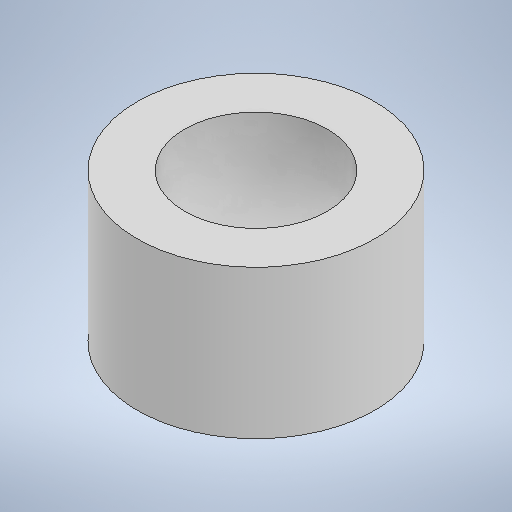
# Autodesk Inventor part: Test1
Saved by Autodesk Inventor 2026.2 (Build 302298010, 298A)
## iProperties
Created: 2026-05-09
Part Number: Test1
Material: Generic
Document SubType Name: Modeling
Designer: piete
Density: 1 g/cm^3
Appearance: Default
Author: piete
Autodesk Inventor part; units mm, degrees
ref_plane "YZ Plane" through (0, 0, 0) normal (1, 0, 0) x (0, 1, 0)
ref_plane "XZ Plane" through (0, 0, 0) normal (0, 1, 0) x (-1, 0, 0)
ref_plane "XY Plane" through (0, 0, 0) normal (0, 0, 1) x (1, 0, 0)
sketch "Sketch1" plane through (0, 0, 0) normal (0, 1, 0) x (-1, 0, 0)
  circle A0 centre (0, 0) radius 20
  dimension "d0" = 40
  constraints: 1 centre point, 1 coincident
  measures "d0" diameter of A0
extrude "Extrusion1" add sketch "Sketch1" along normal blind 25
sketch "Sketch2" plane through (0, 0, 0) normal (1, 0, 0) x (0, 1, 0)
  line L0 (25, -20) -> (25, 20) projected
  line L1 (25, 0) -> (25, -12)
  line L2 (25, -12) -> (25, 12)
  circle A0 centre (25, 12) radius 12.5
  circle A1 centre (25, -12) radius 12.5
  circle A2 centre (21.5, 0) radius 12.5
  line L3 (39.3814, 0) -> (3.1668, 0)
  line L4 (-7.8763, 0) -> (47.2577, 0) projected
  point P0 (0, 0)
  point P1 (34, 0)
  point P2 (9, 0)
  dimension "d5" = 25
  dimension "d6" = 25
  dimension "d3" = 12
  dimension "d4" = 24
  dimension "d7" = 25
  dimension "d8" = 36.2146
  dimension "d9" = 3.1668
  dimension "d10" = 12
  constraints: 6 end point, 2 coincident, 2 point on line, 1 centre point, 1 horizontal, 1 midpoint, 6 other
  measures "d3" distance of L1.start L1.end
  measures "d4" distance of L1.end L2.end
  measures "d7" diameter of A2
  measures "d8" distance of L3.start L3.end
  measures "d9" distance of point (0, 0) L3.end
  measures "d10" distance from line of L1.end L3
revolve "Revolution1" cut sketch "Sketch2" angle 360 about axis through (0, -10, 0) along (0, 1, 0) picked at (21.3864, 4.5774) picked at (25.8062, 7.8367) contours L3 A1 L0 | L0 A1 L3 | L3 A2 A0 | A0 A2 L0 A1 | A1 L0 A2 A0 | A0 A2 L3
body "Solid1"
